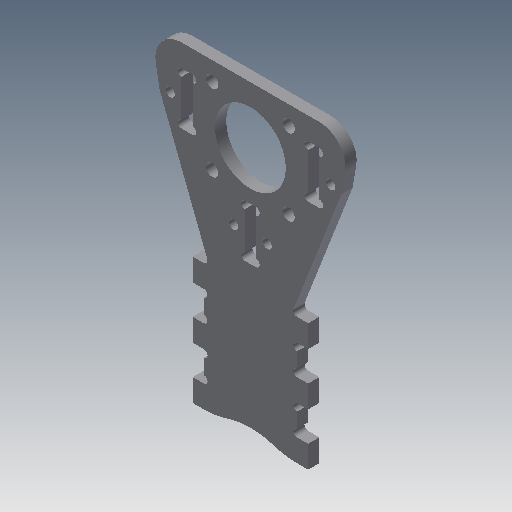
# Autodesk Inventor part: スライダベアリングハウジング
Saved by Autodesk Inventor 2019.4 (Build 234330000, 330)
## iProperties
Created: 2018-08-09
Part Number: スライダベアリングハウジング
Material: 一般
Document SubType Name: Modeling
Designer: Owner
Density: 1 g/cm^3
Appearance: 既定
Mass: 7.00911 g
Surface Area: 62.7617 cm^2
Volume: 7.00911 cm^3
Author: Owner
Autodesk Inventor part; units mm, degrees
ref_plane "YZ Plane" through (0, 0, 0) normal (1, 0, 0) x (0, 1, 0)
ref_plane "XZ Plane" through (0, 0, 0) normal (0, 1, 0) x (-1, 0, 0)
ref_plane "XY Plane" through (0, 0, 0) normal (0, 0, 1) x (1, 0, 0)
sketch "スケッチ1" plane through (0, -85.3303, 0) normal (0, 0, 1) x (1, 0, 0)
  circle A0 centre (0, 85.3303) radius 5 construction
  line L0 (10.253, 75.0773) -> (-10.253, 75.0773) construction
  line L1 (-10.253, 75.0773) -> (-10.253, 95.5834) construction
  line L2 (-10.253, 95.5834) -> (10.253, 95.5834) construction
  line L3 (10.253, 95.5834) -> (10.253, 75.0773) construction
  line L4 (10.253, 75.0773) -> (-10.253, 95.5834) construction
  line L5 (-10.253, 75.0773) -> (10.253, 95.5834) construction
  circle A1 centre (-10.253, 95.5834) radius 1.65
  circle A2 centre (-10.253, 75.0773) radius 1.65
  circle A3 centre (10.253, 75.0773) radius 1.65
  circle A4 centre (10.253, 95.5834) radius 1.65
  circle A5 centre (0, 85.3303) radius 9.5
  line L6 (-15.5, 52.3303) -> (-12.5, 52.3303)
  line L7 (-12.5, 46.3303) -> (-15.5, 46.3303)
  line L8 (-15.5, 46.3303) -> (-15.5, 52.3303)
  line L9 (-15.5, 38.3303) -> (-12.5, 38.3303)
  line L10 (-12.5, 32.3303) -> (-15.5, 32.3303)
  line L11 (-15.5, 32.3303) -> (-15.5, 38.3303)
  line L12 (-15.5, 24.3303) -> (-12.5, 24.3303)
  line L13 (-12.5, 18.3303) -> (-15.5, 18.3303)
  line L14 (-15.5, 18.3303) -> (-15.5, 24.3303)
  arc A6 (-12.5, 24.3303) -> (-12.5, 26.3303) centre (-12.5, 25.3303) ccw
  arc A7 (-12.5, 30.3303) -> (-12.5, 32.3303) centre (-12.5, 31.3303) ccw
  arc A8 (-12.5, 38.3303) -> (-12.5, 40.3303) centre (-12.5, 39.3303) ccw
  arc A9 (-12.5, 44.3303) -> (-12.5, 46.3303) centre (-12.5, 45.3303) ccw
  line L15 (-12.5, 44.3303) -> (-12.5, 40.3303)
  line L16 (-12.5, 30.3303) -> (-12.5, 26.3303)
  arc A10 (-12.5, 52.3303) -> (-11.5677, 53.692) centre (-12.5, 53.3303) ccw
  line L17 (-18.5, 100.5834) -> (0, 100.5834)
  line L18 (0, 100.5834) -> (0, 94.8303)
  line L19 (5, 15.3303) -> (-5, 15.3303) projected
  line L20 (-5, 15.3303) -> (-5, 18.6303) projected
  line L21 (5, 18.6303) -> (-5, 18.6303) projected
  line L22 (5, 15.3303) -> (5, 18.6303) projected
  arc A11 (0, 20.3336) -> (-6.25, 19.3319) centre (0, 0.3336) ccw
  line L23 (0, 20.3336) -> (0, 75.8303)
  arc A12 (-12.5, 18.3303) -> (-6.25, 19.3319) centre (-12.5, 38.3303) ccw
  line L24 (-18.5, 94.5834) -> (-15.5, 94.5834)
  line L25 (-15.5, 92.5834) -> (-15.5, 82.5834)
  line L26 (-15.5, 80.5834) -> (-18.5, 80.5834)
  line L27 (-18.5, 82.5834) -> (-18.5, 92.5834)
  arc A13 (-18.5, 94.5834) -> (-18.5, 92.5834) centre (-18.5, 93.5834) ccw
  arc A14 (-18.5, 82.5834) -> (-18.5, 80.5834) centre (-18.5, 81.5834) ccw
  arc A15 (-15.5, 80.5834) -> (-15.5, 82.5834) centre (-15.5, 81.5834) ccw
  arc A16 (-15.5, 92.5834) -> (-15.5, 94.5834) centre (-15.5, 93.5834) ccw
  circle A17 centre (-21.5, 87.5834) radius 1.25
  arc A18 (-24.4541, 87.0604) -> (-24.2968, 86.4981) centre (-21.5, 87.5834) ccw
  line L28 (-25.3928, 92.3631) -> (-24.4541, 87.0604)
  line L29 (-24.2968, 86.4981) -> (-11.5677, 53.692)
  arc A19 (-18.5, 100.5834) -> (-25.3928, 92.3631) centre (-18.5, 93.5834) ccw
  line L30 (0, 58.3303) -> (-1.5, 58.3303)
  line L31 (-1.5, 60.3303) -> (-1.5, 70.3303)
  line L32 (-1.5, 72.3303) -> (0, 72.3303)
  arc A20 (-1.5, 72.3303) -> (-1.5, 70.3303) centre (-1.5, 71.3303) ccw
  arc A21 (-1.5, 60.3303) -> (-1.5, 58.3303) centre (-1.5, 59.3303) ccw
  circle A22 centre (-4.5, 65.3303) radius 1.25
  point P0 (0, 85.3303)
  point P1 (-15.5, 87.5834)
  point P2 (-1.5, 65.3303)
  dimension "d0" = 29
  dimension "d1" = 3.3
  dimension "d4" = 360
  dimension "d6" = 19
  dimension "d7" = 15.5
  dimension "d8" = 33
  dimension "d9" = 8
  dimension "d10" = 6
  dimension "d11" = 8
  dimension "d12" = 3
  dimension "d13" = 1
  dimension "d16" = 6
  dimension "d17" = 20
  dimension "d19" = 20
  dimension "d24" = 15.5
  dimension "d26" = 3
  dimension "d27" = 2
  dimension "d28" = 14
  dimension "d31" = 18.5
  dimension "d32" = 5
  dimension "d33" = 2.5
  dimension "d34" = 3
  dimension "d35" = 6
  dimension "d36" = 6
  dimension "d37" = 14
  dimension "d38" = 1.5
  dimension "d39" = 2.5
  dimension "d40" = 3
  dimension "d41" = 20
  constraints: 58 end point, 34 point on circle, 26 point on line, 22 centre point, 9 equal radius, 8 parallel, 8 tangent, 7 horizontal, 7 perpendicular, 6 midpoint, 4 vertical alignment, 3 coincident, 2 equal length, 2 horizontal alignment, 2 vertical, 1 collinear, 1 line through centre, 9 other
  measures "d0" distance of L0.start L1.end
  measures "d1" diameter of A1
  measures "d6" diameter of A5
  measures "d7" distance from line of point (0, 85.33) L8
  measures "d8" distance from line of point (0, 85.33) L6
  measures "d9" distance between parallel lines of L9 L7
  measures "d10" distance of L7.end L6.start
  measures "d11" distance between parallel lines of L12 L10
  measures "d12" distance from line of L6.end L8
  measures "d13" radius of A6
  measures "d16" distance of L13.end L12.start
  measures "d17" radius of A11
  measures "d19" radius of A12
  measures "d24" distance between parallel lines of L18 L25
  measures "d26" distance of L24.start L24.end
  measures "d27" diameter of A13
  measures "d28" distance between parallel lines of L26 L24
  measures "d31" distance of L17.start L17.end
  measures "d32" distance from line of L1.end L17
  measures "d33" diameter of A17
  measures "d34" distance from line of L27 A17.centre
  measures "d35" diameter of A18
  measures "d36" distance between parallel lines of L17 L24
  measures "d37" distance between parallel lines of L30 L32
  measures "d38" distance between parallel lines of L23 L31
  measures "d39" diameter of A22
  measures "d40" distance from line of L31 A22.centre
  measures "d41" vertical distance of point (0, 85.33) point (-1.5, 65.33)
extrude "押し出し2" add sketch "スケッチ1" along normal blind 3 contours A5 L23 L32 A20 L31 A21 L30 A11 A12 L13 L14 L12 A6 L16 A7 L10 L11 L9 A8 L15 A9 L7 L8 L6 A10 L29 A18 L28 A19 L17 L18
mirror "ミラー2" about plane through (0, -13, 0) normal (1, 0, 0) of "押し出し2"
equation "\"d11\" = d9"
equation "\"d37\" = d28"
